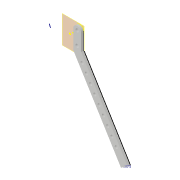
# Autodesk Inventor part: CollectorArmWithAngle
Saved by Autodesk Inventor 2018 (Build 220112000, 112)
## iProperties
Created: 2018-12-09
Part Number: CollectorArmWithAngle
Material: Generic
Document SubType Name: Modeling
Designer: ball
Density: 1 g/cm^3
Appearance: Default
Author: ball
Autodesk Inventor part; units mm, degrees
ref_plane "YZ Plane" through (0, 0, 0) normal (1, 0, 0) x (0, 1, 0)
ref_plane "XZ Plane" through (0, 0, 0) normal (0, 1, 0) x (-1, 0, 0)
ref_plane "XY Plane" through (0, 0, 0) normal (0, 0, 1) x (1, 0, 0)
sketch "Sketch1" plane through (0, 0, 0) normal (0, 0, 1) x (1, 0, 0)
  arc A0 (6.0118, 7.7827) -> (6.4404, 9.2521) centre (8, 8) ccw construction
  arc A1 (7.7827, -6.0118) -> (9.2521, -6.4404) centre (8, -8) ccw construction
  circle A2 centre (8, 8) radius 1.9939 construction
  circle A3 centre (8, -8) radius 1.9939 construction
  line L0 (6.0061, 8) -> (6.0061, -8) construction
  line L1 (1.9277, 2.1329) -> (2.8194, -0.5629) construction
  arc A4 (1.9277, 2.1329) -> (2.8194, -0.5629) centre (0, 0) ccw construction
  line L2 (9.9939, 8) -> (6.0061, 8) construction
  line L3 (6.0061, 8) -> (6.0061, -8) construction
  line L4 (6.0061, -8) -> (9.9939, -8) construction
  line L5 (9.9939, -8) -> (9.9939, 8) construction
  arc A5 (12.7621, 7.9367) -> (3.2375, 8) centre (8, 8) ccw construction
  line L6 (8, 8) -> (3.2375, 8) construction
  line L7 (8, 8) -> (12.7625, 8) construction
  line L8 (12.7625, 10.7686) -> (3.2375, 10.7686) construction
  line L9 (3.2375, 10.7686) -> (3.2375, -14.5363) construction
  line L10 (3.2375, -10.7686) -> (12.7625, -10.7686) construction
  line L11 (12.7625, -11.6614) -> (12.7625, 10.7686) construction
  line L12 (12.7625, 8) -> (12.7625, -11.6614) construction
  line L13 (3.2375, 8) -> (3.2375, -14.5363) construction
  line L14 (125.2938, -2.5112) -> (119.3124, -4.6433) construction
  line L15 (120.3686, -7.6063) -> (119.3124, -4.6433) construction
  circle A6 centre (64.263, -105.1393) radius 2 construction
  circle A7 centre (0, 0) radius 1.9939 construction
  line L16 (64.263, -105.1393) -> (0, 0) construction
  line L17 (0, 0) -> (-1.7037, -1.0359) construction
  line L18 (0, 0) -> (1.9939, 0) construction
  line L19 (0, 0) -> (1.7037, 1.0359) construction
  line L20 (64.263, -105.1393) -> (62.5541, -106.1783) construction
  line L21 (64.263, -105.1393) -> (66.263, -105.1393) construction
  line L22 (64.263, -105.1393) -> (65.9719, -104.1002) construction
  line L23 (1.7037, 1.0359) -> (65.9719, -104.1002) construction
  line L24 (65.9719, -104.1002) -> (62.5591, -106.1865) construction
  line L25 (62.5591, -106.1865) -> (-1.7091, -1.0504) construction
  line L26 (-1.7091, -1.0504) -> (1.7037, 1.0359) construction
  line L27 (-5.5766, -0.1174) -> (61.6261, -110.0539) construction
  line L28 (61.6261, -110.0539) -> (69.8394, -105.0332) construction
  line L29 (69.8394, -105.0332) -> (0.7437, 8) construction
  line L30 (2.6367, 4.9033) -> (-5.5766, -0.1174) construction
  line L31 (64.263, -105.1393) -> (68.3721, -102.633) construction
  line L32 (12.7625, -11.6614) -> (68.3721, -102.633) construction
  line L33 (64.263, -105.1393) -> (60.1589, -107.6537) construction
  line L34 (68.3721, -102.633) -> (60.1589, -107.6537) construction
  line L35 (60.1589, -107.6537) -> (3.2375, -14.5363) construction
  arc A8 (25.7824, -64.2706) -> (22.8, -65.3296) centre (24.3335, -64.9192) ccw construction
  circle A9 centre (43.9887, -120.2705) radius 1.5 construction
  circle A10 centre (43.9887, -120.2705) radius 60.325 construction
  circle A11 centre (34.3115, -56.1364) radius 1.778 construction
  circle A12 centre (8, 8) radius 4.7625
  line L36 (12.7625, -11.6614) -> (3.2375, -14.5363)
  line L37 (3.2375, -14.5363) -> (60.1589, -107.6537)
  line L38 (60.1589, -107.6537) -> (68.3721, -102.633)
  line L39 (68.3721, -102.633) -> (12.7625, -11.6614)
  circle A13 centre (34.3115, -56.1364) radius 1.778
  circle A14 centre (13.9136, -22.7595) radius 1.778
  circle A15 centre (19.013, -31.1037) radius 1.778
  circle A16 centre (24.1123, -39.4479) radius 1.778
  circle A17 centre (29.2117, -47.7921) radius 1.778
  circle A18 centre (39.4103, -64.4804) radius 1.778
  circle A19 centre (44.5097, -72.8246) radius 1.778
  circle A20 centre (49.609, -81.1688) radius 1.778
  circle A21 centre (54.7084, -89.513) radius 1.778
  circle A22 centre (8, -8) radius 1.9939
  circle A23 centre (8, 8) radius 1.9939
  point P0 (0, 0)
  dimension "d1" = 3.9878
  dimension "d0" = 3.9878
  dimension "d3" = 4.7625
  dimension "d4" = 180
  dimension "d5" = 2.7686
  dimension "d6" = 3.9878
  dimension "d7" = 148.7
  dimension "d8" = 148.7
  dimension "d9" = 2.8131
  dimension "d11" = 3.556
  dimension "d98" = 3.9878
  dimension "d99" = 3.9878
  constraints: 78 end point, 21 centre point, 14 point on line, 12 point on circle, 9 coincident, 8 parallel, 7 perpendicular, 4 horizontal, 3 collinear, 3 equal length, 1 concentric, 1 horizontal alignment, 1 tangent, 1 vertical, 36 other
  measures "d0" diameter of A2
  measures "d3" radius of A5
  measures "d4" angle of L6 L7
  measures "d5" distance between parallel lines of L5 L11
  measures "d6" diameter of A7
  measures "d7" angle of L17 L18
  measures "d8" angle of L20 L21
  measures "d9" distance between parallel lines of L25 L27
  measures "d11" diameter of A11
  measures "d98" diameter of A22
  measures "d99" diameter of A23
extrude "Extrusion1" add sketch "Sketch1" along normal blind 3.175 contours A12 | A23
ref_plane "Work Plane1" through (0, 0, 0) normal (0, 0, 1) x (1, 0, 0)
sketch "Sketch2" plane through (0, 0, 0) normal (0, 0, 1) x (1, 0, 0)
  circle A0 centre (8, 8) radius 4.7625 projected
  line L0 (12.7625, 8) -> (3.2375, 8)
  line L1 (3.2375, 8) -> (3.2375, -14.5363)
  line L2 (3.2375, -14.5363) -> (12.7625, -14.5363)
  line L3 (12.7625, -14.5363) -> (12.7625, 8)
  line L4 (3.2375, -14.5363) -> (60.325, -107.95)
  line L5 (60.325, -107.95) -> (68.4525, -102.9831)
  line L6 (68.4525, -102.9831) -> (11.365, -9.5694)
  line L7 (11.365, -9.5694) -> (3.2375, -14.5363)
  point P0 (0, 0)
  dimension "d14" = 9.525
  constraints: 16 end point, 4 parallel, 2 perpendicular, 1 horizontal, 1 horizontal alignment, 1 other
  measures "d14" distance of L5.end L4.end
extrude "Extrusion2" add sketch "Sketch2" along normal blind 3.175 contours L3 L6 L7 L1 A0 | A0 L0 | L6 L5 L4 L2 L3 | L3 L2 L7 L6 picked at (6.8117, 6.9473)
hole "Hole1" at (34.311, -56.1362, 0) direction (0, 0, 1) diameter 3.556 end through all
hole "Hole2" at (49.6089, -81.1686, 0) direction (0, 0, 1) diameter 3.556 end through all
hole "Hole3" at (44.509, -72.8243, 0) direction (0, 0, 1) diameter 3.556 end through all
hole "Hole4" at (54.7081, -89.5129, 0) direction (0, 0, 1) diameter 3.556 end through all
hole "Hole5" at (39.4103, -64.4805, 0) direction (0, 0, 1) diameter 3.556 end through all
hole "Hole6" at (29.2063, -47.787, 0) direction (0, 0, 1) diameter 3.556 end through all
hole "Hole7" at (24.11, -39.4457, 0) direction (0, 0, 1) diameter 3.556 end through all
hole "Hole8" at (19.0131, -31.1028, 0) direction (0, 0, 1) diameter 3.556 end through all
hole "Hole9" at (13.917, -22.7563, 0) direction (0, 0, 1) diameter 3.556 end through all
sketch "Sketch3" plane through (60.325, -107.95, 0) normal (-0.8532764, -0.5214589, 0) x (0, 0, 1)
  point P0 (0, 123.5682)
sketch "Sketch4" plane through (0, 0, 3.175) normal (0, 0, 1) x (1, 0, 0)
  spline S0 degree 3 poles (-25.2788, -2.0557) (-25.3112, -1.9605) (-25.3341, -1.8916) (-25.3588, -1.8128) (-25.3613, -1.8009) (-25.3441, -1.8374) (-25.3155, -1.9119) (-25.2521, -2.0803) (-25.2004, -2.2209) (-25.0761, -2.5633) (-25.0055, -2.7599) (-24.8596, -3.169) (-24.7792, -3.3953) (-24.6138, -3.8659) (-24.5358, -4.0898) (-24.3927, -4.5052) (-24.3289, -4.6925) (-24.2382, -4.9635) (-24.1921, -5.103) (-24.1408, -5.2711) (-24.1321, -5.3068) (-24.1428, -5.2998) (-24.1636, -5.2531) (-24.2396, -5.0631) (-24.2901, -4.9305) (-24.3621, -4.7401) (-24.4003, -4.6379) (-24.4829, -4.4155) (-24.5269, -4.296) (-24.5725, -4.1714) knots 0.000001 0.000001 0.000001 0.000001 0.060915 0.060915 0.118968 0.118968 0.203575 0.203575 0.324675 0.324675 0.441995 0.441995 0.548902 0.548902 0.648718 0.648718 0.748605 0.748605 0.82225 0.82225 0.878767 0.878767 0.938156 0.938156 1.008318 1.008318 1.073219 1.073219 1.138691 1.138691 1.138691 1.138691
  point P0 (0, 0)
  constraints: 4 other
sketch "Sketch5" plane through (0, 0, 0) normal (0, 0, -1) x (-1, 0, 0)
  arc A0 (-9.9544, 7.5753) -> (-9.6822, 9.0817) centre (-8, 8) ccw projected
  arc A1 (-7.5753, -9.9544) -> (-9.0817, -9.6822) centre (-8, -8) ccw
  circle A2 centre (-8, 8) radius 2
  circle A3 centre (-8, -8) radius 2
  point P0 (0, 0)
  constraints: 3 centre point, 2 coincident, 2 concentric, 2 point on circle, 4 other
hole "Hole10" at (8, -8, 0) direction (0, 0, 1) diameter 3.9878 end through all
hole "Hole11" at (8, 8, 0) direction (0, 0, 1) diameter 3.9878 end through all
body "Solid1"
